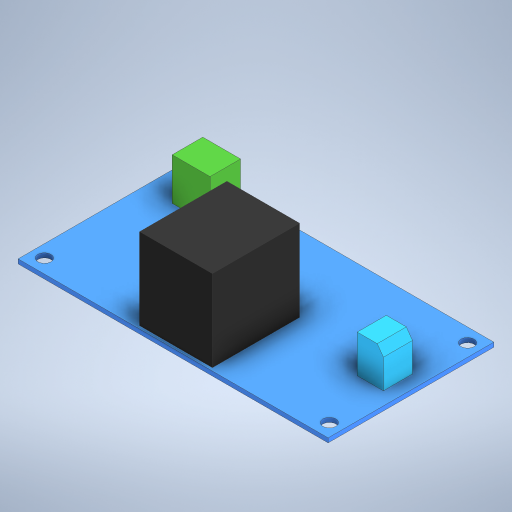
# Autodesk Inventor part: AC-DC컨버터
Saved by Autodesk Inventor 2023 (Build 270158000, 158)
## iProperties
Created: 2022-08-18
Part Number: AC-DC컨버터
Material: 일반
Document SubType Name: Modeling
Designer: user
Density: 1 g/cm^3
Appearance: 기본값
Author: user
Autodesk Inventor part; units mm, degrees
ref_plane "YZ Plane" through (0, 0, 0) normal (1, 0, 0) x (0, 1, 0)
ref_plane "XZ Plane" through (0, 0, 0) normal (0, 1, 0) x (-1, 0, 0)
ref_plane "XY Plane" through (0, 0, 0) normal (0, 0, 1) x (1, 0, 0)
sketch "스케치1" plane through (0, 0, 0) normal (0, 1, 0) x (-1, 0, 0)
  line L0 (-53.3, 28.5) -> (53.3, 28.5)
  line L1 (53.3, 28.5) -> (53.3, -28.5)
  line L2 (53.3, -28.5) -> (-53.3, -28.5)
  line L3 (-53.3, -28.5) -> (-53.3, 28.5)
  line L4 (-53.3, 28.5) -> (53.3, -28.5) construction
  line L5 (53.3, 28.5) -> (-53.3, -28.5) construction
  circle A0 centre (49, 23.75) radius 2.25
  line L6 (0, 0) -> (18.7645, 0)
  line L7 (0, 0) -> (0, -10.3185)
  circle A1 centre (-49, 23.75) radius 2.25
  circle A2 centre (49, -23.75) radius 2.25
  circle A3 centre (-49, -23.75) radius 2.25
  dimension "d0" = 106.6
  dimension "d1" = 57
  dimension "d2" = 4.5
  dimension "d3" = 47.5
  dimension "d4" = 98
  constraints: 16 end point, 4 centre point, 3 symmetric about line, 2 horizontal, 2 midpoint, 2 parallel, 1 perpendicular, 1 vertical, 3 other
  measures "d0" distance of L1.end L2.end
  measures "d1" distance of L0.end L1.end
  measures "d2" diameter of A0
  measures "d3" distance of A2.centre A0.centre
  measures "d4" distance of A3.centre A2.centre
extrude "돌출1" add sketch "스케치1" along normal blind 1.5
sketch "스케치2" plane through (0, 1.5, 0) normal (0, 1, 0) x (1, 0, 0)
  line L0 (-43.3, 14.5) -> (-30.3, 14.5)
  line L1 (-30.3, 14.5) -> (-30.3, 25)
  line L2 (-30.3, 25) -> (-43.3, 25)
  line L3 (-43.3, 25) -> (-43.3, 14.5)
  line L4 (-43.3, 14.5) -> (-30.3, 25) construction
  line L5 (-30.3, 14.5) -> (-43.3, 25) construction
  line L6 (-53.3, 28.5) -> (-53.3, -28.5) projected
  line L7 (53.3, 28.5) -> (-53.3, 28.5) projected
  point P0 (0, 0)
  point P1 (-36.8, 19.75)
  dimension "d7" = 10.5
  dimension "d8" = 13
  dimension "d9" = 10
  dimension "d10" = 3.5
  constraints: 12 end point, 2 midpoint, 2 parallel, 1 horizontal, 1 perpendicular
  measures "d7" distance of L2.end L0.start
  measures "d8" distance of L1.end L2.end
  measures "d9" distance between parallel lines of L6 L3
  measures "d10" distance between parallel lines of L7 L2
extrude "돌출2" add sketch "스케치2" along normal blind 14.5
sketch "스케치3" plane through (0, 1.5, 0) normal (0, 1, 0) x (1, 0, 0)
  line L0 (12.5, -27.5) -> (-12.5, -27.5)
  line L1 (-12.5, -27.5) -> (-12.5, 2.5)
  line L2 (-12.5, 2.5) -> (12.5, 2.5)
  line L3 (12.5, 2.5) -> (12.5, -27.5)
  line L4 (12.5, -27.5) -> (-12.5, 2.5) construction
  line L5 (-12.5, -27.5) -> (12.5, 2.5) construction
  line L6 (-53.3, -28.5) -> (53.3, -28.5) projected
  point P0 (0, 0)
  point P1 (0, -12.5)
  dimension "d13" = 25
  dimension "d14" = 30
  dimension "d15" = 16
  constraints: 12 end point, 2 midpoint, 2 parallel, 1 horizontal, 1 perpendicular, 1 vertical alignment
  measures "d13" distance of L1.end L2.end
  measures "d14" distance of L0.end L1.end
  measures "d15" distance from line of L6 point (0, -12.5)
extrude "돌출3" add sketch "스케치3" along normal blind 28
sketch "스케치4" plane through (0, 0, 0) normal (0, 0, 1) x (1, 0, 0)
  line L0 (-53.3, 1.5) -> (53.3, 1.5) projected
  line L1 (48.8, 1.5) -> (48.8, 11.5)
  line L2 (48.8, 11.5) -> (46.6994, 14.5)
  line L3 (46.6994, 14.5) -> (39.8, 14.5)
  line L4 (39.8, 14.5) -> (39.8, 1.5)
  point P0 (0, 0)
  dimension "d18" = 9
  dimension "d19" = 145
  dimension "d20" = 13
  dimension "d21" = 4.5
  dimension "d22" = 10
  constraints: 8 end point, 2 perpendicular, 2 point on line, 1 vertical
  measures "d18" distance of L4.end L1.start
  measures "d19" angle of L1 L2
  measures "d20" distance of L3.end L4.end
  measures "d21" distance of L0.end L1.start
  measures "d22" distance of L1.start L1.end
extrude "돌출4" add sketch "스케치4" along normal mid plane 10
